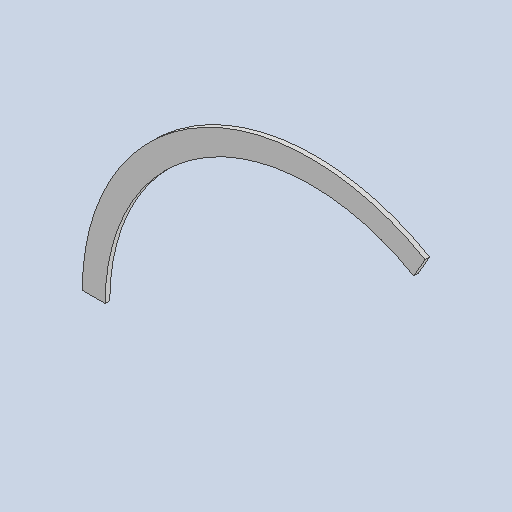
# Autodesk Inventor part: треть-кольцо
Saved by Autodesk Inventor 2024.2 (Build 282272000, 272)
## iProperties
Created: 2024-04-17
Part Number: треть-кольцо
Material: Generic
Document SubType Name: Sheet Metal
Designer: admin
Density: 1 g/cm^3
Sheet Metal Rule: Default_mm
Appearance: Default
Flat Pattern Width: 10 cm
Flat Pattern Length: 15 cm
Flat Pattern Area: 150 cm^2
Sheet Metal Width: 100,000 mm
Sheet Metal Length: 150,000 mm
Sheet Metal Area: 15000,000 mm^2
Author: admin
Autodesk Inventor part; units mm, degrees
ref_plane "YZ Plane" through (0, 0, 0) normal (1, 0, 0) x (0, 1, 0)
ref_plane "XZ Plane" through (0, 0, 0) normal (0, 1, 0) x (-1, 0, 0)
ref_plane "XY Plane" through (0, 0, 0) normal (0, 0, 1) x (1, 0, 0)
sketch "Sketch1" plane through (0, 0, 0) normal (0, 0, 1) x (1, 0, 0)
  circle A0 centre (0, 0) radius 100
  circle A1 centre (0, 0) radius 90
  line L0 (-100, 0) -> (0, 0)
  line L1 (0, 0) -> (50, 86.6025)
  point P0 (45, 77.9423)
  point P1 (-90, 0)
  dimension "d0" = 200
  dimension "d1" = 10
  dimension "d2" = 120
  measures "d0" diameter of A0
  measures "d1" radial gap between concentric circles of A0 A1
  measures "d2" angle of L1 L0
extrude "Plate1" add sketch "Sketch1" along normal blind 2 contours L1 A1 L0 A0 picked at (-96.3423, 4.6391)
equation "\"d0\" = Внешний_диам_тарелки"
equation "\"d3\" = Thickness"
equation "\"BendRadius\" = Thickness"
equation "\"BendReliefWidth\" = Thickness"
equation "\"BendReliefDepth\" = 0.5 * Thickness"
equation "\"CornerReliefSize\" = 4 * Thickness"
equation "\"MinimumRemnant\" = 2 * Thickness"
equation "\"TransitionRadius\" = BendRadius"
equation "\"JacobiRadiusSize\" = BendRadius"
equation "\"GapSize\" = Thickness"
equation "\"Внешний_диам_тарелки\" = 200"
equation "\"Thickness\" = 2"
body "Solid1"
